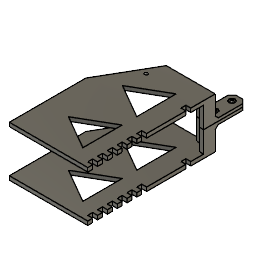
Ball Launcher 3000 (Autodesk Fusion 360 design; units mm, degrees)
Autodesk Fusion 360 part; units mm, degrees
note: some values were not read from the file. Set by a fixed rule: which sketch regions a step uses.
sketch "Sketch1" plane through (0, 0, 0) normal (0, 0, 1) x (1, 0, 0)
  line L0 (40, 65) -> (-40, 65)
  line L1 (-40, 65) -> (-40, -65)
  line L2 (-40, -65) -> (40, -65)
  line L3 (40, -65) -> (40, 65)
  line L4 (40, 65) -> (-40, -65) construction
  line L5 (-40, 65) -> (40, -65) construction
  circle A0 centre (-13.0359, 47.7417) radius 1.7
  line L6 (-16.5, 49.7417) -> (4, 85.2487)
  line L7 (4, 85.2487) -> (0.5359, 87.2487)
  line L8 (0.5359, 87.2487) -> (-19.9641, 51.7417)
  line L9 (-19.9641, 51.7417) -> (-16.5, 49.7417)
  line L10 (-19.9641, 51.7417) -> (-69.4641, -33.9948)
  line L11 (-16.5, 49.7417) -> (-66, -35.9948)
  line L12 (-66, -35.9948) -> (-69.4641, -33.9948)
  circle A1 centre (12, 81.23) radius 20
  circle A2 centre (12, 81.23) radius 8
  line L13 (4, 85.2487) -> (4, 65)
  line L14 (-40, 61) -> (40, 61)
  circle A3 centre (32, 90) radius 1.7
  circle A4 centre (32, 72.46) radius 1.7
  line L15 (40, 65) -> (40, 97)
  line L16 (40, 97) -> (25, 97)
  line L17 (25, 97) -> (25, 65)
  circle A5 centre (32, 90) radius 3.1
  circle A6 centre (32, 72.46) radius 3.1
  line L18 (0, 2.5) -> (0, 20)
  line L19 (-10, 65) -> (-40, 13.0385)
  line L20 (20, -10) -> (20, -50)
  line L21 (20, -50) -> (-14.641, -30)
  line L22 (-14.641, -30) -> (20, -10)
  line L23 (-14.641, 25) -> (20, 45)
  line L24 (20, 5) -> (-14.641, 25)
  line L25 (20, 45) -> (20, 5)
  line L26 (25, 65) -> (25, 61)
  line L27 (40, 61) -> (36, 61)
  line L28 (36, 61) -> (36, 53)
  line L29 (36, 53) -> (40, 53)
  line L30 (40, 53) -> (40, 61)
  line L31 (40, 40) -> (35, 40)
  line L32 (35, 40) -> (35, 35)
  line L33 (35, 35) -> (40, 35)
  line L34 (40, 35) -> (40, 40)
  line L35 (35, -55) -> (40, -55)
  line L36 (40, -55) -> (40, -60)
  line L37 (40, -60) -> (35, -60)
  line L38 (35, -60) -> (35, -55)
  line L39 (35, -45) -> (40, -45)
  line L40 (35, -50) -> (35, -45)
  line L41 (40, -50) -> (35, -50)
  line L42 (35, -35) -> (40, -35)
  line L43 (35, -40) -> (35, -35)
  line L44 (40, -40) -> (35, -40)
  line L45 (35, -25) -> (40, -25)
  line L46 (35, -30) -> (35, -25)
  line L47 (40, -30) -> (35, -30)
  line L48 (35, -15) -> (40, -15)
  line L49 (35, -20) -> (35, -15)
  line L50 (40, -20) -> (35, -20)
  line L51 (35, -5) -> (40, -5)
  line L52 (35, -10) -> (35, -5)
  line L53 (40, -10) -> (35, -10)
  dimension "d1" = 80
  dimension "d2" = 130
  dimension "d5" = 3.4
  dimension "d8" = 41
  dimension "d9" = 4
  dimension "d10" = 4
  dimension "d13" = 99
  dimension "d14" = 40
  dimension "d15" = 16
  dimension "d17" = 8
  dimension "d18" = 4
  dimension "d19" = 3.4
  dimension "d20" = 3.4
  dimension "d21" = 17.54
  dimension "d22" = 8.77
  dimension "d23" = 20
  dimension "d24" = 8
  dimension "d25" = 15
  dimension "d26" = 32
  dimension "d29" = 6.2
  dimension "d30" = 6.2
  dimension "d42" = 30
  dimension "d43" = 40
  dimension "d44" = 2
  dimension "d45" = 30
  dimension "d54" = 60
  dimension "d55" = 60
  dimension "d56" = 40
  dimension "d57" = 15
  dimension "d58" = 20
  dimension "d59" = 60
  dimension "d60" = 60
  dimension "d61" = 40
  dimension "d62" = 15
  dimension "d63" = 20
  dimension "d64" = 7
  dimension "d65" = 4
  dimension "d66" = 8
  dimension "d67" = 5
  dimension "d68" = 21
  dimension "d69" = 5
  dimension "d71" = 5
  dimension "d72" = 5
  dimension "d73" = 5
  dimension "d76" = 0
  dimension "d77" = 10
  constraint horizontal L0
  constraint perpendicular L0 L1
  constraint parallel L0 L2
  constraint parallel L1 L3
  constraint coincident L4 origin
  constraint coincident L5 origin
  constraint perpendicular L6 L7
  constraint perpendicular L7 L8
  constraint perpendicular L8 L9
  constraint coincident A0.centre L9
  constraint perpendicular L9 L10
  constraint perpendicular L9 L11
  constraint perpendicular L10 L12
  constraint concentric A1 A2
  constraint coincident L0 L13.end
  constraint perpendicular L0 L13
  constraint coincident L1 L14.start
  constraint coincident L3 L14.end
  constraint perpendicular L3 L14
  constraint vertical A3.centre A4.centre
  constraint coincident L0 L3.end
  constraint perpendicular L0 L15
  constraint perpendicular L15 L16
  constraint coincident L0 L17.end
  constraint perpendicular L0 L17
  constraint concentric A3 A5
  constraint concentric A4 A6
  constraint coincident L0 L19.start
  constraint coincident L1 L19.end
  constraint parallel L10 L19
  constraint perpendicular L14 L20
  constraint parallel L3 L25
  constraint coincident L14 L26.end
  constraint perpendicular L14 L26
  constraint horizontal L27
  constraint vertical L28
  constraint horizontal L29
  constraint vertical L30
  constraint horizontal L31
  constraint vertical L32
  constraint horizontal L33
  constraint vertical L34
  constraint coincident L3 L31.start
  constraint horizontal L35
  constraint vertical L36
  constraint horizontal L37
  constraint vertical L38
  constraint coincident L3 L36.end
  measures "d1" distance of L1.end L2.end
  measures "d2" distance of L0.end L1.end
  measures "d5" diameter of A0
  measures "d8" distance of L7.end L8.end
  measures "d9" distance of L6.end L7.end
  measures "d10" distance of A0.centre L6
  measures "d13" distance of L8.end L10.end
  measures "d14" diameter of A1
  measures "d15" diameter of A2
  measures "d17" distance of A1.centre L13
  measures "d18" distance of L0 L14
  measures "d19" diameter of A3
  measures "d20" diameter of A4
  measures "d21" distance of A3.centre A4.centre
  measures "d22" vertical distance of A1.centre A4.centre
  measures "d23" horizontal distance of A1.centre A3.centre
  measures "d24" distance of A3.centre L15
  measures "d25" distance of L15.end L16.end
  measures "d26" distance of L0.start L15.end
  measures "d29" diameter of A5
  measures "d30" diameter of A6
  measures "d42" angle of L11 L18
  measures "d43" distance of origin L15
  measures "d44" distance of L11 L19
  measures "d45" distance of L1 L19.start
  measures "d54" angle of L20 L21
  measures "d55" angle of L20 L22
  measures "d56" distance of L20.start L20.end
  measures "d57" distance of L2 L20.end
  measures "d58" distance of L3 L20
  measures "d59" angle of L24 L25
  measures "d60" angle of L23 L25
  measures "d61" distance of L24.start L23.end
  measures "d62" distance of L20.start L24.start
  measures "d63" distance of L3 L25
  measures "d64" distance of L16 A3.centre
  measures "d65" distance of L28.end L29.end
  measures "d66" distance of L27.end L28.end
  measures "d67" distance of L31.end L32.end
  measures "d68" distance of L14 L31
  measures "d69" distance of L31.start L31.end
  measures "d71" distance of L35.start L37.end
  measures "d72" distance of L36.end L37.end
  measures "d73" distance of L2 L37
extrude "Extrude1" add sketch "Sketch1" along normal blind 3 contours L0 A1 L15 L16 L17 A5 A6 | A1 L17 A5 A6 | A1 A6 | A1 A6 | A1 A5 | A1 A5 makes body 1
extrude "Extrude2" cut sketch "Sketch1" along normal blind 5 and the other way blind -2 contours A1 A6 | A1 A6 | A1 A5 | A1 A5 bodies 1
extrude "Extrude3" add sketch "Sketch1" along normal blind 25.6 contours L0 L3 L14 L26 L27 | L3 L14 L27 L28 L29 L30 bodies 1
extrude "Extrude4" add sketch "Sketch1" along normal blind 25.6 and the other way blind -21.6 contours L0 L3 L14 L26 L27 | L0 L6 A1 L14 L26 | L3 L14 L27 L28 L29 L30 | L0 A1 | L1 L2 L3 L6 L11 L14 L28 L29 L31 L32 L33 L35 L37 L38 L39 L40 L41 L42 L43 L44 L45 L46 L47 L48 L49 L50 L51 L52 L53 | L0 L6 L14 L19 | L6 L9 L14 L19 | L1 L9 L11 L19 bodies 1
chamfer "Chamfer1" distance 4 angle 45 2 edges at (40, 97, 1.5) (25, 97, 1.5) on bodies 1
chamfer "Chamfer1" distance 3 angle 45 1 edges at (32.5, 65, 3) on bodies 1
mirror "Mirror1" about plane through (0, 0, 0) normal (0, 0, 1) of bodies 1 makes body 2
equation "d17 = d15 / 2"
equation "d21 = ( ( 14.38 + 20.7 ) / 2 ) * 1 mm"
equation "d22 = d21 / 2"
equation "d35 = ( ( 60 + 2 - 18.8 ) / 2 ) * 1 mm + 4 mm"
equation "d39 = -25.6 mm + 4 mm"
equation "d43 = d1 / 2"
equation "d55 = d54"
equation "d60 = d54"
equation "d62 = d57"
equation "d63 = d58"
